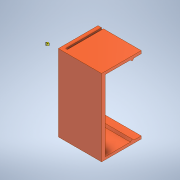
# Autodesk Inventor part: usbHubCaseTopPowerSide
Saved by Autodesk Inventor 2021.2 (Build 252289000, 289)
## iProperties
Created: 2021-02-17
Part Number: usbHubCaseTopPowerSide
Material: PC/ABS Plastic
Document SubType Name: Modeling
Designer: robst
Density: 0.357273 g/cm^3
Appearance: Smooth - Light Orange
Author: robst
Autodesk Inventor part; units mm, degrees
ref_plane "YZ Plane" through (0, 0, 0) normal (1, 0, 0) x (0, 1, 0)
ref_plane "XZ Plane" through (0, 0, 0) normal (0, 1, 0) x (-1, 0, 0)
ref_plane "XY Plane" through (0, 0, 0) normal (0, 0, 1) x (1, 0, 0)
sketch "Sketch1" plane through (0, 0, 0) normal (0, 0, 1) x (1, 0, 0)
  line L0 (-15.24, -26.9875) -> (15.24, -26.9875)
  line L1 (15.24, -26.9875) -> (15.24, 26.9875)
  line L2 (15.24, 26.9875) -> (-15.24, 26.9875)
  line L3 (-15.24, 26.9875) -> (-15.24, -26.9875)
  line L4 (-15.24, -26.9875) -> (15.24, 26.9875) construction
  line L5 (15.24, -26.9875) -> (-15.24, 26.9875) construction
  point P0 (0, 0)
  dimension "d0" = 53.975
  dimension "d1" = 30.48
  constraints: 12 end point, 2 midpoint, 2 parallel, 1 horizontal, 1 perpendicular
  measures "d0" distance of L2.end L0.start
  measures "d1" distance of L1.end L2.end
extrude "Extrusion1" add sketch "Sketch1" against normal blind 2.54
sketch "Sketch8" plane through (0, 0, -2.54) normal (0, 0, -1) x (-1, 0, 0)
  line L0 (-15.24, 26.9875) -> (-15.24, -26.9875) projected
  line L1 (15.24, -26.9875) -> (15.24, 26.9875) projected
  line L2 (-15.24, 26.9875) -> (15.24, 26.9875)
  line L3 (15.24, 26.9875) -> (15.24, 25.0825)
  line L4 (15.24, 25.0825) -> (-15.24, 25.0825)
  line L5 (-15.24, 25.0825) -> (-15.24, 26.9875)
  line L6 (-15.24, -26.9875) -> (15.24, -26.9875)
  line L7 (15.24, -26.9875) -> (15.24, -25.0825)
  line L8 (15.24, -25.0825) -> (-15.24, -25.0825)
  line L9 (-15.24, -25.0825) -> (-15.24, -26.9875)
  line L10 (15.24, 25.0825) -> (12.7, 25.0825)
  line L11 (12.7, 25.0825) -> (12.7, 12.8905)
  line L12 (12.7, 12.8905) -> (15.24, 12.8905)
  line L13 (15.24, 12.8905) -> (15.24, 25.0825)
  line L14 (15.24, -25.0825) -> (12.7, -25.0825)
  line L15 (12.7, -25.0825) -> (12.7, -12.8905)
  line L16 (12.7, -12.8905) -> (15.24, -12.8905)
  line L17 (15.24, -12.8905) -> (15.24, -25.0825)
  point P0 (0, 0)
  point P1 (15.24, -12.8905)
  point P2 (15.24, 12.8905)
  dimension "d32" = 1.905
  dimension "d33" = 1.905
  dimension "d34" = 2.54
  dimension "d35" = 12.192
  dimension "d36" = 12.192
  dimension "d37" = 2.54
  constraints: 32 end point, 8 parallel, 4 horizontal, 4 perpendicular, 2 point on line
  measures "d32" distance between parallel lines of L4 L2
  measures "d33" distance between parallel lines of L8 L6
  measures "d34" distance between parallel lines of L11 L1
  measures "d35" distance between parallel lines of L12 L4
  measures "d36" distance between parallel lines of L16 L8
  measures "d37" distance between parallel lines of L1 L15
extrude "Extrusion7" add sketch "Sketch8" along normal blind 25.4 contours L2 L1 L4 L0 | L8 L1 L6 L0 | L4 L1 L12 L11 | L15 L16 L1 L8
sketch "Sketch10" plane through (0, 0, -2.54) normal (0, 0, -1) x (-1, 0, 0)
  line L0 (12.7, 25.0825) -> (12.7, 12.8905) projected
  line L1 (12.7, 12.8905) -> (15.24, 12.8905)
  line L2 (15.24, 12.8905) -> (15.24, -12.8905)
  line L3 (15.24, -12.8905) -> (12.7, -12.8905)
  line L4 (12.7, -12.8905) -> (12.7, 12.8905)
  point P0 (0, 0)
  constraints: 8 end point, 2 parallel, 1 horizontal, 1 perpendicular
extrude "Extrusion8" add sketch "Sketch10" along normal blind 6.096
sketch "Sketch11" plane through (15.24, -26.9875, 0) normal (1, 0, 0) x (0, 0, -1)
  line L0 (2.54, 1.905) -> (27.94, 1.905) projected
  line L1 (2.54, 52.07) -> (27.94, 52.07) projected
  line L2 (20.32, 1.905) -> (21.59, 3.175)
  line L3 (21.59, 3.175) -> (22.86, 1.905)
  line L4 (2.54, 1.905) -> (27.94, 1.905) projected
  line L5 (27.94, 14.097) -> (27.94, 1.905) projected
  line L6 (20.32, 1.905) -> (22.86, 1.905)
  line L7 (0, 26.9875) -> (27.94, 26.9875) construction
  line L8 (2.54, 52.07) -> (27.94, 52.07)
  line L9 (20.32, 52.07) -> (21.59, 50.8)
  line L10 (21.59, 50.8) -> (22.86, 52.07)
  point P0 (22.86, 1.905)
  dimension "d42" = 90
  dimension "d43" = 135
  dimension "d44" = 1.27
  dimension "d45" = 6.35
  constraints: 14 end point, 3 point on line, 3 symmetric about line, 1 collinear, 1 horizontal
  measures "d42" angle of L3 L2
  measures "d43" angle of L3 L0
  measures "d44" distance from line of L2.end L0
  measures "d45" distance from line of L2.end L5
extrude "Extrusion9" add sketch "Sketch11" against normal up to surface (27.94 mm away)
sketch "Sketch12" plane through (-15.24, 26.9875, 0) normal (0, 1, 0) x (1, 0, 0)
  line L0 (2.54, 2.54) -> (2.54, 20.32) projected
  line L1 (2.54, 22.86) -> (2.54, 27.94) projected
  line L2 (2.54, 27.94) -> (3.81, 27.94)
  line L3 (3.81, 27.94) -> (3.81, 2.54)
  line L4 (3.81, 2.54) -> (2.54, 2.54)
  line L5 (2.54, 2.54) -> (2.54, 27.94)
  point P0 (15.24, 0)
  point P1 (2.54, 22.86)
  point P2 (2.54, 20.32)
  dimension "d48" = 1.27
  constraints: 8 end point, 2 parallel, 1 horizontal, 1 perpendicular
  measures "d48" distance between parallel lines of L1 L3
extrude "Extrusion10" cut sketch "Sketch12" against normal through all
sketch "Sketch13" plane through (0, 0, -2.54) normal (0, 0, -1) x (-1, 0, 0)
  line L0 (-15.24, 26.9875) -> (15.24, 26.9875) construction
  line L1 (-1.27, 26.9875) -> (-1.27, -28.2825) construction
  line L2 (-15.24, 25.0825) -> (-15.24, -25.0825) construction
  spline S0 degree 2 poles (-5.2014, -4.6721) (-4.9544, -4.6721) (-4.5098, -4.8481) (-4.3555, -5.0055) knots 0 0 0 1 2 2 2
  spline S1 degree 2 poles (-4.3555, -5.0055) (-4.1609, -5.2031) (-3.9603, -5.7373) (-3.9603, -6.1448) knots 0 0 0 1 2 2 2
  line L3 (-3.9603, -6.1448) -> (-3.9603, -6.574)
  line L4 (-3.9603, -6.574) -> (-2.54, -6.574)
  line L5 (-2.54, -6.574) -> (-2.54, -7.0804)
  line L6 (-2.54, -7.0804) -> (-6.35, -7.0804)
  line L7 (-6.35, -7.0804) -> (-6.35, -6.1232)
  spline S2 degree 2 poles (-6.35, -6.1232) (-6.35, -5.7836) (-6.2388, -5.3081) (-6.1123, -5.126) knots 0 0 0 1 2 2 2
  spline S3 degree 2 poles (-6.1123, -5.126) (-5.9671, -4.9129) (-5.5195, -4.6721) (-5.2014, -4.6721) knots 0 0 0 1 2 2 2
  spline S4 degree 2 poles (-5.186, -5.2001) (-5.3836, -5.2001) (-5.6738, -5.3359) (-5.7665, -5.4748) knots 0 0 0 1 2 2 2
  spline S5 degree 2 poles (-5.7665, -5.4748) (-5.8467, -5.5953) (-5.9116, -5.9164) (-5.9116, -6.1541) knots 0 0 0 1 2 2 2
  line L8 (-5.9116, -6.1541) -> (-5.9116, -6.574)
  line L9 (-5.9116, -6.574) -> (-4.3925, -6.574)
  line L10 (-4.3925, -6.574) -> (-4.3925, -6.2282)
  spline S6 degree 2 poles (-4.3925, -6.2282) (-4.3925, -5.9194) (-4.4913, -5.5397) (-4.621, -5.4162) knots 0 0 0 1 2 2 2
  spline S7 degree 2 poles (-4.621, -5.4162) (-4.7352, -5.3019) (-5.0038, -5.2001) (-5.186, -5.2001) knots 0 0 0 1 2 2 2
  line L11 (-6.35, -1.4271) -> (-2.54, -2.7393)
  line L12 (-2.54, -2.7393) -> (-2.54, -3.2858)
  line L13 (-2.54, -3.2858) -> (-6.35, -4.598)
  line L14 (-6.35, -4.598) -> (-6.35, -4.0546)
  line L15 (-6.35, -4.0546) -> (-3.1853, -2.9987)
  line L16 (-3.1853, -2.9987) -> (-6.35, -1.9427)
  line L17 (-6.35, -1.9427) -> (-6.35, -1.4271)
  line L18 (-3.9757, 0.2679) -> (-3.9757, -1.1739)
  line L19 (-3.9757, -1.1739) -> (-4.4388, -1.1739)
  line L20 (-4.4388, -1.1739) -> (-4.4388, 0.2679)
  line L21 (-4.4388, 0.2679) -> (-3.9757, 0.2679)
  spline S8 degree 2 poles (-4.445, 3.1455) (-3.4199, 3.1455) (-2.4597, 2.5496) (-2.4597, 1.929) knots 0 0 0 1 2 2 2
  spline S9 degree 2 poles (-2.4597, 1.929) (-2.4597, 1.2992) (-3.4385, 0.7095) (-4.4419, 0.7095) knots 0 0 0 1 2 2 2
  spline S10 degree 2 poles (-4.4419, 0.7095) (-5.4731, 0.7095) (-6.4272, 1.3054) (-6.4272, 1.929) knots 0 0 0 1 2 2 2
  spline S11 degree 2 poles (-6.4272, 1.929) (-6.4272, 2.5558) (-5.4392, 3.1455) (-4.445, 3.1455) knots 0 0 0 1 2 2 2
  spline S12 degree 2 poles (-3.2841, 2.491) (-3.4724, 2.5651) (-4.0529, 2.6268) (-4.445, 2.6268) knots 0 0 0 1 2 2 2
  spline S13 degree 2 poles (-4.445, 2.6268) (-4.8371, 2.6268) (-5.4145, 2.5651) (-5.609, 2.4879) knots 0 0 0 1 2 2 2
  spline S14 degree 2 poles (-5.609, 2.4879) (-5.8035, 2.4107) (-6.0042, 2.1421) (-6.0042, 1.929) knots 0 0 0 1 2 2 2
  spline S15 degree 2 poles (-6.0042, 1.929) (-6.0042, 1.716) (-5.8035, 1.4412) (-5.6028, 1.3609) knots 0 0 0 1 2 2 2
  spline S16 degree 2 poles (-5.6028, 1.3609) (-5.4083, 1.2837) (-4.8155, 1.2282) (-4.4419, 1.2282) knots 0 0 0 1 2 2 2
  spline S17 degree 2 poles (-4.4419, 1.2282) (-4.0405, 1.2282) (-3.5033, 1.2776) (-3.2934, 1.3578) knots 0 0 0 1 2 2 2
  spline S18 degree 2 poles (-3.2934, 1.3578) (-3.0958, 1.4319) (-2.8827, 1.7067) (-2.8827, 1.929) knots 0 0 0 1 2 2 2
  spline S19 degree 2 poles (-2.8827, 1.929) (-2.8827, 2.139) (-3.0834, 2.4138) (-3.2841, 2.491) knots 0 0 0 1 2 2 2
  spline S20 degree 2 poles (-5.9888, 4.6615) (-5.9888, 4.5225) (-5.9208, 4.2478) (-5.8683, 4.115) knots 0 0 0 1 2 2 2
  spline S21 degree 2 poles (-5.8683, 4.115) (-5.8159, 3.9915) (-5.7047, 3.8093) (-5.6553, 3.7383) knots 0 0 0 1 2 2 2
  line L22 (-5.6553, 3.7383) -> (-5.6553, 3.7074)
  line L23 (-5.6553, 3.7074) -> (-6.1956, 3.7074)
  spline S22 degree 2 poles (-6.1956, 3.7074) (-6.2852, 3.8742) (-6.4303, 4.4454) (-6.4303, 4.7016) knots 0 0 0 1 2 2 2
  spline S23 degree 2 poles (-6.4303, 4.7016) (-6.4303, 4.961) (-6.3253, 5.3469) (-6.2141, 5.5044) knots 0 0 0 1 2 2 2
  spline S24 degree 2 poles (-6.2141, 5.5044) (-6.0937, 5.6711) (-5.7448, 5.844) (-5.5102, 5.844) knots 0 0 0 1 2 2 2
  spline S25 degree 2 poles (-5.5102, 5.844) (-5.1953, 5.844) (-4.7198, 5.4303) (-4.658, 5.1401) knots 0 0 0 1 2 2 2
  line L24 (-4.658, 5.1401) -> (-4.621, 5.1401)
  spline S26 degree 2 poles (-4.621, 5.1401) (-4.5963, 5.2605) (-4.4851, 5.5353) (-4.374, 5.6526) knots 0 0 0 1 2 2 2
  spline S27 degree 2 poles (-4.374, 5.6526) (-4.2659, 5.7699) (-3.9201, 5.9181) (-3.67, 5.9181) knots 0 0 0 1 2 2 2
  spline S28 degree 2 poles (-3.67, 5.9181) (-3.4138, 5.9181) (-2.9784, 5.7421) (-2.8117, 5.5816) knots 0 0 0 1 2 2 2
  spline S29 degree 2 poles (-2.8117, 5.5816) (-2.6388, 5.4148) (-2.4597, 4.9425) (-2.4597, 4.643) knots 0 0 0 1 2 2 2
  spline S30 degree 2 poles (-2.4597, 4.643) (-2.4597, 4.3558) (-2.5987, 3.7939) (-2.6944, 3.6025) knots 0 0 0 1 2 2 2
  line L25 (-2.6944, 3.6025) -> (-3.2347, 3.6025)
  line L26 (-3.2347, 3.6025) -> (-3.2347, 3.6395)
  spline S31 degree 2 poles (-3.2347, 3.6395) (-3.1174, 3.8001) (-2.9012, 4.3435) (-2.9012, 4.6121) knots 0 0 0 1 2 2 2
  spline S32 degree 2 poles (-2.9012, 4.6121) (-2.9012, 4.7695) (-3, 5.0845) (-3.1143, 5.1895) knots 0 0 0 1 2 2 2
  spline S33 degree 2 poles (-3.1143, 5.1895) (-3.2285, 5.2913) (-3.5002, 5.3994) (-3.7071, 5.3994) knots 0 0 0 1 2 2 2
  spline S34 degree 2 poles (-3.7071, 5.3994) (-3.9139, 5.3994) (-4.1826, 5.279) (-4.2597, 5.1709) knots 0 0 0 1 2 2 2
  spline S35 degree 2 poles (-4.2597, 5.1709) (-4.3369, 5.0629) (-4.3956, 4.7695) (-4.3956, 4.5966) knots 0 0 0 1 2 2 2
  line L27 (-4.3956, 4.5966) -> (-4.3956, 4.3805)
  line L28 (-4.3956, 4.3805) -> (-4.8186, 4.3805)
  line L29 (-4.8186, 4.3805) -> (-4.8186, 4.5503)
  spline S36 degree 2 poles (-4.8186, 4.5503) (-4.8186, 4.8931) (-5.1459, 5.3253) (-5.4577, 5.3253) knots 0 0 0 1 2 2 2
  spline S37 degree 2 poles (-5.4577, 5.3253) (-5.6028, 5.3253) (-5.8097, 5.2142) (-5.8714, 5.1246) knots 0 0 0 1 2 2 2
  spline S38 degree 2 poles (-5.8714, 5.1246) (-5.9363, 5.0289) (-5.9888, 4.7942) (-5.9888, 4.6615) knots 0 0 0 1 2 2 2
  spline S39 degree 2 poles (1.1798, -10.6897) (1.4268, -10.6897) (1.8714, -10.8657) (2.0258, -11.0231) knots 0 0 0 1 2 2 2
  spline S40 degree 2 poles (2.0258, -11.0231) (2.2203, -11.2207) (2.421, -11.7549) (2.421, -12.1624) knots 0 0 0 1 2 2 2
  line L30 (2.421, -12.1624) -> (2.421, -12.5916)
  line L31 (2.421, -12.5916) -> (3.8412, -12.5916)
  line L32 (3.8412, -12.5916) -> (3.8412, -13.0979)
  line L33 (3.8412, -13.0979) -> (0.0312, -13.0979)
  line L34 (0.0312, -13.0979) -> (0.0312, -12.1408)
  spline S41 degree 2 poles (0.0312, -12.1408) (0.0312, -11.8012) (0.1424, -11.3257) (0.269, -11.1435) knots 0 0 0 1 2 2 2
  spline S42 degree 2 poles (0.269, -11.1435) (0.4141, -10.9305) (0.8618, -10.6897) (1.1798, -10.6897) knots 0 0 0 1 2 2 2
  spline S43 degree 2 poles (1.1952, -11.2176) (0.9976, -11.2176) (0.7074, -11.3535) (0.6148, -11.4924) knots 0 0 0 1 2 2 2
  spline S44 degree 2 poles (0.6148, -11.4924) (0.5345, -11.6128) (0.4696, -11.9339) (0.4696, -12.1717) knots 0 0 0 1 2 2 2
  line L35 (0.4696, -12.1717) -> (0.4696, -12.5916)
  line L36 (0.4696, -12.5916) -> (1.9887, -12.5916)
  line L37 (1.9887, -12.5916) -> (1.9887, -12.2458)
  spline S45 degree 2 poles (1.9887, -12.2458) (1.9887, -11.937) (1.8899, -11.5573) (1.7602, -11.4338) knots 0 0 0 1 2 2 2
  spline S46 degree 2 poles (1.7602, -11.4338) (1.646, -11.3195) (1.3774, -11.2176) (1.1952, -11.2176) knots 0 0 0 1 2 2 2
  spline S47 degree 2 poles (2.4117, -7.8955) (3.1342, -7.8955) (3.9215, -8.5902) (3.9215, -9.1706) knots 0 0 0 1 2 2 2
  spline S48 degree 2 poles (3.9215, -9.1706) (3.9215, -9.7665) (3.1095, -10.4488) (2.4117, -10.4488) knots 0 0 0 1 2 2 2
  spline S49 degree 2 poles (2.4117, -10.4488) (1.6954, -10.4488) (0.9019, -9.7449) (0.9019, -9.1706) knots 0 0 0 1 2 2 2
  spline S50 degree 2 poles (0.9019, -9.1706) (0.9019, -8.5902) (1.6923, -7.8955) (2.4117, -7.8955) knots 0 0 0 1 2 2 2
  spline S51 degree 2 poles (2.4117, -8.3925) (1.8559, -8.3925) (1.3156, -8.797) (1.3156, -9.1706) knots 0 0 0 1 2 2 2
  spline S52 degree 2 poles (1.3156, -9.1706) (1.3156, -9.5442) (1.8559, -9.9517) (2.4117, -9.9517) knots 0 0 0 1 2 2 2
  spline S53 degree 2 poles (2.4117, -9.9517) (2.952, -9.9517) (3.5078, -9.5442) (3.5078, -9.1706) knots 0 0 0 1 2 2 2
  spline S54 degree 2 poles (3.5078, -9.1706) (3.5078, -8.8001) (2.9613, -8.3925) (2.4117, -8.3925) knots 0 0 0 1 2 2 2
  line L38 (0.9822, -3.9373) -> (3.8412, -4.6628)
  line L39 (3.8412, -4.6628) -> (3.8412, -5.1074)
  line L40 (3.8412, -5.1074) -> (1.6367, -5.8052)
  line L41 (1.6367, -5.8052) -> (3.8412, -6.4999)
  line L42 (3.8412, -6.4999) -> (3.8412, -6.9414)
  line L43 (3.8412, -6.9414) -> (0.9822, -7.6732)
  line L44 (0.9822, -7.6732) -> (0.9822, -7.173)
  line L45 (0.9822, -7.173) -> (3.1959, -6.6666)
  line L46 (3.1959, -6.6666) -> (0.9822, -5.9905)
  line L47 (0.9822, -5.9905) -> (0.9822, -5.5922)
  line L48 (0.9822, -5.5922) -> (3.1959, -4.8975)
  line L49 (3.1959, -4.8975) -> (0.9822, -4.422)
  line L50 (0.9822, -4.422) -> (0.9822, -3.9373)
  spline S55 degree 2 poles (3.9061, -2.2731) (3.9061, -2.9585) (3.1373, -3.7119) (2.4271, -3.7119) knots 0 0 0 1 2 2 2
  spline S56 degree 2 poles (2.4271, -3.7119) (1.7294, -3.7119) (0.9019, -2.9801) (0.9019, -2.3904) knots 0 0 0 1 2 2 2
  spline S57 degree 2 poles (0.9019, -2.3904) (0.9019, -2.1249) (1.0563, -1.7142) (1.2199, -1.563) knots 0 0 0 1 2 2 2
  spline S58 degree 2 poles (1.2199, -1.563) (1.3836, -1.4086) (1.8559, -1.2449) (2.1987, -1.2449) knots 0 0 0 1 2 2 2
  line L51 (2.1987, -1.2449) -> (2.4611, -1.2449)
  line L52 (2.4611, -1.2449) -> (2.4611, -3.224)
  spline S59 degree 2 poles (2.4611, -3.224) (2.9582, -3.224) (3.4862, -2.7239) (3.4862, -2.2793) knots 0 0 0 1 2 2 2
  spline S60 degree 2 poles (3.4862, -2.2793) (3.4862, -2.1218) (3.4151, -1.8161) (3.3596, -1.6926) knots 0 0 0 1 2 2 2
  spline S61 degree 2 poles (3.3596, -1.6926) (3.2978, -1.563) (3.1898, -1.3839) (3.1403, -1.3252) knots 0 0 0 1 2 2 2
  line L53 (3.1403, -1.3252) -> (3.1403, -1.2974)
  line L54 (3.1403, -1.2974) -> (3.6652, -1.2974)
  spline S62 degree 2 poles (3.6652, -1.2974) (3.6992, -1.3808) (3.798, -1.634) (3.8258, -1.7328) knots 0 0 0 1 2 2 2
  spline S63 degree 2 poles (3.8258, -1.7328) (3.8659, -1.8717) (3.9061, -2.1002) (3.9061, -2.2731) knots 0 0 0 1 2 2 2
  spline S64 degree 2 poles (2.0937, -1.7142) (1.8992, -1.7204) (1.6151, -1.8007) (1.5194, -1.8779) knots 0 0 0 1 2 2 2
  spline S65 degree 2 poles (1.5194, -1.8779) (1.4113, -1.9612) (1.2971, -2.2237) (1.2971, -2.4182) knots 0 0 0 1 2 2 2
  spline S66 degree 2 poles (1.2971, -2.4182) (1.2971, -2.6096) (1.4113, -2.8782) (1.5225, -2.9894) knots 0 0 0 1 2 2 2
  spline S67 degree 2 poles (1.5225, -2.9894) (1.6367, -3.0975) (1.9115, -3.2086) (2.0937, -3.224) knots 0 0 0 1 2 2 2
  line L55 (2.0937, -3.224) -> (2.0937, -1.7142)
  line L56 (1.4978, 0.7589) -> (1.4978, 0.7342)
  spline S68 degree 2 poles (1.4978, 0.7342) (1.4824, 0.6786) (1.4762, 0.5582) (1.4762, 0.4748) knots 0 0 0 1 2 2 2
  spline S69 degree 2 poles (1.4762, 0.4748) (1.4762, 0.2803) (1.646, -0.1026) (1.8127, -0.2755) knots 0 0 0 1 2 2 2
  line L57 (1.8127, -0.2755) -> (3.8412, -0.2755)
  line L58 (3.8412, -0.2755) -> (3.8412, -0.7571)
  line L59 (3.8412, -0.7571) -> (0.9822, -0.7571)
  line L60 (0.9822, -0.7571) -> (0.9822, -0.2755)
  line L61 (0.9822, -0.2755) -> (1.4083, -0.2755)
  spline S70 degree 2 poles (1.4083, -0.2755) (1.1736, -0.013) (0.9822, 0.3791) (0.9822, 0.5643) knots 0 0 0 1 2 2 2
  spline S71 degree 2 poles (0.9822, 0.5643) (0.9822, 0.6384) (0.9883, 0.7125) (0.9976, 0.7589) knots 0 0 0 1 2 2 2
  line L62 (0.9976, 0.7589) -> (1.4978, 0.7589)
  spline S72 degree 2 poles (3.9091, 3.868) (3.9091, 3.4543) (3.7362, 2.8738) (3.6127, 2.6175) knots 0 0 0 1 2 2 2
  line L63 (3.6127, 2.6175) -> (2.9767, 2.6175)
  line L64 (2.9767, 2.6175) -> (2.9767, 2.6546)
  spline S73 degree 2 poles (2.9767, 2.6546) (3.2114, 2.9047) (3.4707, 3.5376) (3.4707, 3.8309) knots 0 0 0 1 2 2 2
  spline S74 degree 2 poles (3.4707, 3.8309) (3.4707, 4.2508) (3.1218, 4.68) (2.8347, 4.68) knots 0 0 0 1 2 2 2
  spline S75 degree 2 poles (2.8347, 4.68) (2.6062, 4.68) (2.3222, 4.4546) (2.2511, 4.2107) knots 0 0 0 1 2 2 2
  spline S76 degree 2 poles (2.2511, 4.2107) (2.2017, 4.0347) (2.1338, 3.7414) (2.0782, 3.5222) knots 0 0 0 1 2 2 2
  spline S77 degree 2 poles (2.0782, 3.5222) (2.0258, 3.3246) (1.8683, 3.0128) (1.7417, 2.8923) knots 0 0 0 1 2 2 2
  spline S78 degree 2 poles (1.7417, 2.8923) (1.6151, 2.775) (1.2755, 2.6453) (1.0532, 2.6453) knots 0 0 0 1 2 2 2
  spline S79 degree 2 poles (1.0532, 2.6453) (0.5901, 2.6453) (-0.0367, 3.3678) (-0.0367, 3.9267) knots 0 0 0 1 2 2 2
  spline S80 degree 2 poles (-0.0367, 3.9267) (-0.0367, 4.2478) (0.0899, 4.8159) (0.2103, 5.0598) knots 0 0 0 1 2 2 2
  line L65 (0.2103, 5.0598) -> (0.8154, 5.0598)
  line L66 (0.8154, 5.0598) -> (0.8154, 5.0227)
  spline S81 degree 2 poles (0.8154, 5.0227) (0.6487, 4.8406) (0.4017, 4.2725) (0.4017, 3.9606) knots 0 0 0 1 2 2 2
  spline S82 degree 2 poles (0.4017, 3.9606) (0.4017, 3.6086) (0.7321, 3.1733) (1.0007, 3.1733) knots 0 0 0 1 2 2 2
  spline S83 degree 2 poles (1.0007, 3.1733) (1.2415, 3.1733) (1.5287, 3.4296) (1.5935, 3.6704) knots 0 0 0 1 2 2 2
  spline S84 degree 2 poles (1.5935, 3.6704) (1.6367, 3.8309) (1.7479, 4.2972) (1.7942, 4.4515) knots 0 0 0 1 2 2 2
  spline S85 degree 2 poles (1.7942, 4.4515) (1.9146, 4.8437) (2.3993, 5.208) (2.7544, 5.208) knots 0 0 0 1 2 2 2
  spline S86 degree 2 poles (2.7544, 5.208) (2.9798, 5.208) (3.4121, 5.0258) (3.5633, 4.8622) knots 0 0 0 1 2 2 2
  spline S87 degree 2 poles (3.5633, 4.8622) (3.7301, 4.68) (3.9091, 4.2169) (3.9091, 3.868) knots 0 0 0 1 2 2 2
  line L67 (3.8412, 6.1775) -> (3.8412, 5.6958)
  line L68 (3.8412, 5.6958) -> (0.9822, 5.6958)
  line L69 (0.9822, 5.6958) -> (0.9822, 6.1775)
  line L70 (0.9822, 6.1775) -> (3.8412, 6.1775)
  line L71 (0.5067, 6.2114) -> (0.5067, 5.6649)
  line L72 (0.5067, 5.6649) -> (0.0065, 5.6649)
  line L73 (0.0065, 5.6649) -> (0.0065, 6.2114)
  line L74 (0.0065, 6.2114) -> (0.5067, 6.2114)
  line L75 (3.8412, 9.0828) -> (3.8412, 8.6012)
  line L76 (3.8412, 8.6012) -> (3.551, 8.6012)
  spline S88 degree 2 poles (3.551, 8.6012) (3.6436, 8.49) (3.7671, 8.3264) (3.8196, 8.2152) knots 0 0 0 1 2 2 2
  spline S89 degree 2 poles (3.8196, 8.2152) (3.869, 8.1133) (3.9215, 7.8941) (3.9215, 7.749) knots 0 0 0 1 2 2 2
  spline S90 degree 2 poles (3.9215, 7.749) (3.9215, 7.5144) (3.727, 7.1192) (3.5386, 6.9802) knots 0 0 0 1 2 2 2
  spline S91 degree 2 poles (3.5386, 6.9802) (3.3503, 6.8413) (2.7945, 6.6869) (2.4333, 6.6869) knots 0 0 0 1 2 2 2
  spline S92 degree 2 poles (2.4333, 6.6869) (2.0566, 6.6869) (1.5071, 6.8814) (1.3002, 7.0512) knots 0 0 0 1 2 2 2
  spline S93 degree 2 poles (1.3002, 7.0512) (1.1149, 7.2087) (0.9019, 7.6502) (0.9019, 7.8941) knots 0 0 0 1 2 2 2
  spline S94 degree 2 poles (0.9019, 7.8941) (0.9019, 8.1072) (0.9976, 8.4252) (1.0964, 8.6012) knots 0 0 0 1 2 2 2
  line L77 (1.0964, 8.6012) -> (-0.1386, 8.6012)
  line L78 (-0.1386, 8.6012) -> (-0.1386, 9.0828)
  line L79 (-0.1386, 9.0828) -> (3.8412, 9.0828)
  line L80 (3.1465, 8.6012) -> (1.4947, 8.6012)
  spline S95 degree 2 poles (1.4947, 8.6012) (1.4083, 8.4221) (1.3434, 8.138) (1.3434, 7.9744) knots 0 0 0 1 2 2 2
  spline S96 degree 2 poles (1.3434, 7.9744) (1.3434, 7.6039) (1.8992, 7.184) (2.424, 7.184) knots 0 0 0 1 2 2 2
  spline S97 degree 2 poles (2.424, 7.184) (2.9304, 7.184) (3.4645, 7.5051) (3.4645, 7.8602) knots 0 0 0 1 2 2 2
  spline S98 degree 2 poles (3.4645, 7.8602) (3.4645, 8.0485) (3.2916, 8.4313) (3.1465, 8.6012) knots 0 0 0 1 2 2 2
  spline S99 degree 2 poles (3.9061, 11.0218) (3.9061, 10.3363) (3.1373, 9.583) (2.4271, 9.583) knots 0 0 0 1 2 2 2
  spline S100 degree 2 poles (2.4271, 9.583) (1.7294, 9.583) (0.9019, 10.3147) (0.9019, 10.9045) knots 0 0 0 1 2 2 2
  spline S101 degree 2 poles (0.9019, 10.9045) (0.9019, 11.17) (1.0563, 11.5806) (1.2199, 11.7319) knots 0 0 0 1 2 2 2
  spline S102 degree 2 poles (1.2199, 11.7319) (1.3836, 11.8863) (1.8559, 12.0499) (2.1987, 12.0499) knots 0 0 0 1 2 2 2
  line L81 (2.1987, 12.0499) -> (2.4611, 12.0499)
  line L82 (2.4611, 12.0499) -> (2.4611, 10.0708)
  spline S103 degree 2 poles (2.4611, 10.0708) (2.9582, 10.0708) (3.4862, 10.571) (3.4862, 11.0156) knots 0 0 0 1 2 2 2
  spline S104 degree 2 poles (3.4862, 11.0156) (3.4862, 11.1731) (3.4151, 11.4787) (3.3596, 11.6022) knots 0 0 0 1 2 2 2
  spline S105 degree 2 poles (3.3596, 11.6022) (3.2978, 11.7319) (3.1898, 11.911) (3.1403, 11.9696) knots 0 0 0 1 2 2 2
  line L83 (3.1403, 11.9696) -> (3.1403, 11.9974)
  line L84 (3.1403, 11.9974) -> (3.6652, 11.9974)
  spline S106 degree 2 poles (3.6652, 11.9974) (3.6992, 11.9141) (3.798, 11.6609) (3.8258, 11.5621) knots 0 0 0 1 2 2 2
  spline S107 degree 2 poles (3.8258, 11.5621) (3.8659, 11.4232) (3.9061, 11.1947) (3.9061, 11.0218) knots 0 0 0 1 2 2 2
  spline S108 degree 2 poles (2.0937, 11.5806) (1.8992, 11.5744) (1.6151, 11.4942) (1.5194, 11.417) knots 0 0 0 1 2 2 2
  spline S109 degree 2 poles (1.5194, 11.417) (1.4113, 11.3336) (1.2971, 11.0712) (1.2971, 10.8767) knots 0 0 0 1 2 2 2
  spline S110 degree 2 poles (1.2971, 10.8767) (1.2971, 10.6852) (1.4113, 10.4166) (1.5225, 10.3055) knots 0 0 0 1 2 2 2
  spline S111 degree 2 poles (1.5225, 10.3055) (1.6367, 10.1974) (1.9115, 10.0863) (2.0937, 10.0708) knots 0 0 0 1 2 2 2
  line L85 (2.0937, 10.0708) -> (2.0937, 11.5806)
  point P0 (0, 0)
  dimension "d51" = 13.97
  constraints: 2 end point, 2 vertical, 1 point on line
  measures "d51" distance between parallel lines of L1 L2
extrude "Extrusion11" cut sketch "Sketch13" against normal blind 1.27
equation "\"d2\" = usbHolderWallThickness"
equation "\"usbHolderWallThickness\" = 2.54"
equation "\"usbHubWidth\" = 44.45"
equation "\"usbHubDepth\" = 27.432"
equation "\"usbHubLength\" = 109.22"
equation "\"usbHolderWidth\" = 58.42"
equation "\"usbHolderLength\" = usbHubLength + 2 * usbHolderWallThickness"
equation "\"holePatternLength\" = 25.4"
equation "\"holePatternWidth\" = 50.8"
body "Solid1"
